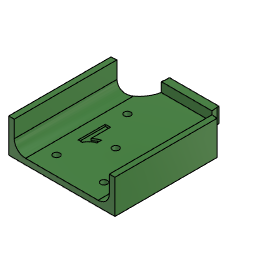
1 - Y Frame Marker (Autodesk Fusion 360 design; units mm, degrees)
Autodesk Fusion 360 part; units mm, degrees
sketch "Profile" plane through (0, 450, 0) normal (0, 1, 0) x (-1, 0, 0)
  line L0 (600, 15) -> (600, 0)
  line L1 (600, 0) -> (650.3, 0)
  line L2 (650.3, 0) -> (650.3, 15)
  line L3 (644.3, 0) -> (606, 0)
  line L4 (597, 15) -> (597, -3)
  line L5 (597, -3) -> (653.3, -3)
  line L6 (653.3, -3) -> (653.3, 15)
  line L7 (597, 15) -> (653.3, 15)
  dimension "d4811" = 50.3
  dimension "d4812" = 15
  dimension "d4813" = 3
  dimension "d4850" = 0
  dimension "d4851" = 0
  dimension "d4852" = 0
  dimension "d4853" = 0
  constraint vertical L0
  constraint perpendicular L0 L1
  constraint perpendicular L1 L2
  constraint equal L0 L2
  constraint midpoint L1 L3
  constraint perpendicular L6 L7
  measures "d4811" distance of L0 L2
  measures "d4812" distance of L1 L2.end
extrude "Extrude1" add sketch "Profile" along normal blind 3
extrude "Extrude2" add sketch "Profile" against normal up to surface (66.2 mm away) contours L0 L1 L2 L3 L4 L5 L6 L7
sketch "Holes and Text" plane through (0, 0, 0) normal (0, 0, 1) x (-1, 0, 0)
  circle A0 centre (637.725, -431.2) radius 1.75
  circle A1 centre (612.575, -431.2) radius 1.75
  circle A2 centre (637.725, -393.6) radius 1.75
  circle A3 centre (612.575, -393.6) radius 1.75
  line L0 (632.575, -420.6) -> (640.075, -420.6) construction
  line L1 (640.075, -420.6) -> (640.075, -400.6) construction
  line L2 (640.075, -400.6) -> (632.575, -400.6) construction
  line L3 (632.575, -400.6) -> (632.575, -420.6) construction
  line L4 (597, -383.8) -> (597, -453)
  line L5 (653.3, -453) -> (597, -453)
  line L6 (653.3, -383.8) -> (653.3, -453)
  arc A4 (612, -453) -> (597, -438) centre (597, -453) ccw
  arc A5 (653.3, -438) -> (638.3, -453) centre (653.3, -453) ccw
  line L7 (637.725, -431.2) -> (612.575, -393.6) construction
  circle A6 centre (625.15, -412.4) radius 1.75
  circle A7 centre (637.725, -431.2) radius 3
  circle A8 centre (612.575, -431.2) radius 3
  circle A9 centre (612.575, -393.6) radius 3
  circle A10 centre (637.725, -393.6) radius 3
  point P0 (597, -453)
  point P1 (653.3, -453)
  dimension "d4818" = 3.5
  dimension "d4819" = 7
  dimension "d4822" = 20
  dimension "d4823" = 20
  dimension "d4824" = 7.5
  dimension "d4825" = 15
  text T0 "1" font "Arial" height 20 bold align ink ink in box 0 x 0 at (632.575, -420.6) x (1, 0) y (0, 1) spacing 1 height is em
  constraint concentric A0 A7
  constraint concentric A1 A8
  constraint concentric A2 A10
  constraint concentric A3 A9
  constraint equal A0 A1
  constraint equal A0 A3
  constraint equal A0 A2
  constraint perpendicular L0 L1
  constraint parallel L0 L2
  constraint parallel L1 L3
  constraint horizontal L2
  constraint coincident P1 L5.start
  constraint coincident P0 L4.end
  constraint coincident L4 A4.end
  constraint coincident L5 A4.start
  constraint coincident L5 A5.end
  constraint coincident L6 A5.start
  constraint equal A4 A5
  constraint coincident A0.centre L7.start
  constraint coincident A3.centre L7.end
  constraint midpoint L7 A6.centre
  constraint equal A2 A6
  measures "d4818" diameter of A0
  measures "d4819" distance of A3.centre L2
  measures "d4822" distance of A1.centre L3
  measures "d4823" distance of L0 L2
  measures "d4824" distance of L1 L3
  measures "d4825" radius of A4
extrude "Extrude3" cut sketch "Holes and Text" along normal up to surface (-3 mm away) and the other way up to surface (-15 mm away) contours A0 | A1 | A2 | A3 | L4 L5 A4 | L5 L6 A5 | A6
extrude "Extrude4" cut 1 faces at (-629.5333, 452.3293, 15) along direction (0, 0, -1) blind 10
fillet "Fillet1" radius 6 2 edges at (-650.3, 411.0515, 0) (-600, 411.0515, 0)
extrude "Extrude5" cut sketch "Holes and Text" against normal blind 1 text T0
extrude "Extrude6" add 1 faces at (-620.7667, 453, 2.3333) along direction (0, 1, 0) blind 1
move_face "OffsetFaces1" offset -0.075 2 faces at (-650.3, 420.1354, 12) (-600, 420.1354, 12)
equation "d4811 = extrusionNarrow"
equation "d4832 = extrusionRadius"
equation "d5478 = -tolerance / 2"
equation "extrusionNarrow = 50.3 mm"
equation "extrusionRadius = 6 mm"
equation "tolerance = 0.15 mm"
